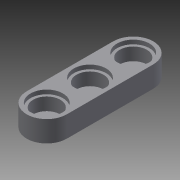
# Autodesk Inventor part: LEGO technic thin liftarm
Saved by Autodesk Inventor 2013 (Build 170138000, 138)
## iProperties
Created: 2013-06-22
Part Number: LEGO technic thin liftarm
Material: Generic
Document SubType Name: Modeling
Designer: Masta
Density: 1 g/cm^3
Author: Masta
Autodesk Inventor part; units mm, degrees
ref_plane "YZ Plane" through (0, 0, 0) normal (1, 0, 0) x (0, 1, 0)
ref_plane "XZ Plane" through (0, 0, 0) normal (0, 1, 0) x (-1, 0, 0)
sketch "Sketch1" plane through (0, 0, 0) normal (0, 0, 1) x (1, 0, 0)
  line L0 (0, 0) -> (1.6, 0) construction
  circle A0 centre (0, 0) radius 2.5
  circle A1 centre (0, 0) radius 3
  arc A2 (0, 3.7) -> (-3.7, 0) centre (0, 0) ccw
  line L1 (0, 0) -> (0, 3.7) construction
  line L2 (0, 3.7) -> (0, 3.7)
  arc A3 (3.7, 0) -> (0, 3.7) centre (0, 0) ccw
  line L3 (0, 0) -> (0, 0) construction
  line L4 (0, 0) -> (-3.7, 0) construction
  line L5 (-3.7, 0) -> (-3.7, -16)
  arc A4 (-3.7, -16) -> (0, -19.7) centre (0, -16) ccw
  line L6 (0, -19.7) -> (0, -19.7)
  arc A5 (0, -19.7) -> (3.7, -16) centre (0, -16) ccw
  line L7 (3.7, -16) -> (3.7, 0)
  dimension "x" = 1.6
  dimension "d1" = 5
  dimension "d2" = 6
  dimension "d3" = 3.7
  dimension "d4" = 0
  dimension "d17" = 16
  constraints: 16 end point, 8 point on circle, 8 tangent, 6 centre point, 3 coincident, 3 parallel, 2 equal radius, 2 horizontal, 2 perpendicular, 1 vertical
  measures "x" distance of L0.start L0.end
  measures "d1" diameter of A0
  measures "d2" diameter of A1
  measures "d3" radius of A2
  measures "d4" distance of L1.end L2.end
  measures "d17" distance of L4.end L5.end
extrude "Extrusion1" add sketch "Sketch1" along normal mid plane 3.9 contours A0 | A1 | A3 L7 A5 A4 L5 A2
extrude "Extrusion2" cut sketch "Sketch1" against normal up to surface (3.9 mm away) from surface at 1.95 contours A0 | A1
extrude "Extrusion3" add sketch "Sketch1" along normal mid plane 2.4 contours A1
pattern_linear "Rectangular Pattern1" count 3 spacing -8 along (0, 1, 0) of "Extrusion2", "Extrusion3"
ref_plane "Work Plane1" through (0, 0, -1.15) normal (0, 0, -1) x (-1, 0, 0)
extrude "Extrusion4" add sketch "Sketch1" along normal up to surface (0.05 mm away) from surface at -1.2 contours A0 | A1 | A3 L7 A5 A4 L5 A2
equation "\"d13\" = 5 * x"
equation "\"d20\" = -5 * x"
body "Solid1"
